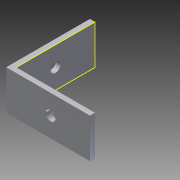
# Autodesk Inventor part: SideSupport
Saved by Autodesk Inventor 2013 (Build 170138000, 138)
## iProperties
Created: 2013-07-15
Part Number: SideSupport
Material: Aluminum 6061
Document SubType Name: Modeling
Designer: root
Density: 1 g/cm^3
Author: root
Autodesk Inventor part; units mm, degrees
ref_plane "YZ Plane" through (0, 0, 0) normal (1, 0, 0) x (0, 1, 0)
ref_plane "XZ Plane" through (0, 0, 0) normal (0, 1, 0) x (-1, 0, 0)
ref_plane "XY Plane" through (0, 0, 0) normal (0, 0, 1) x (1, 0, 0)
sketch "Sketch1" plane through (0, 0, 0) normal (1, 0, 0) x (0, 1, 0)
  line L0 (0, 0) -> (12.7, 0)
  line L1 (12.7, 0) -> (12.7, 25.4)
  line L2 (12.7, 25.4) -> (0, 25.4)
  line L3 (0, 25.4) -> (0, 0)
  dimension "d0" = 25.4
  dimension "d1" = 12.7
  constraints: 8 end point, 2 parallel, 1 horizontal, 1 perpendicular
  measures "d0" distance of L2.end L0.start
  measures "d1" distance of L0.start L0.end
extrude "Extrusion1" add sketch "Sketch1" along normal blind 1.5875
sketch "Sketch2" plane through (1.5875, 0, 0) normal (1, 0, 0) x (0, 0, -1)
  line L0 (0, 0) -> (0, 12.7) projected
  line L1 (0, 12.7) -> (-25.4, 12.7) projected
  line L2 (-25.4, 12.7) -> (-25.4, 0) projected
  line L3 (-25.4, 0) -> (0, 0) projected
sketch "Sketch3" plane through (0, 0, 0) normal (-1, 0, 0) x (0, 0, 1)
  line L0 (25.4, 12.7) -> (26.9875, 12.7)
  line L1 (26.9875, 12.7) -> (26.9875, 0)
  line L2 (26.9875, 0) -> (25.4, 0)
  line L3 (25.4, 0) -> (25.4, 12.7)
  dimension "d4" = 1.5875
  constraints: 8 end point, 2 parallel, 1 horizontal, 1 perpendicular
  measures "d4" distance of L1.end L2.end
extrude "Extrusion2" add sketch "Sketch3" against normal blind 26.9875
sketch "Sketch4" plane through (1.5875, 0, 0) normal (1, 0, 0) x (0, 0, -1)
  line L0 (0, 0) -> (0, 12.7) projected
  line L1 (-25.4, 0) -> (0, 0) projected
  point P0 (-12.7, 6.35)
  dimension "d8" = 6.35
  dimension "d9" = 12.7
  measures "d8" distance from line of L1 point (-12.7, 6.35)
  measures "d9" distance from line of point (-12.7, 6.35) L0
sketch "Sketch5" plane through (26.9875, 12.7, 25.4) normal (0, 0, -1) x (-1, 0, 0)
  line L0 (0, -12.7) -> (0, 0) projected
  line L1 (25.4, -12.7) -> (0, -12.7) projected
  point P0 (26.9875, -12.7)
  point P1 (12.7, -6.35)
  dimension "d10" = 6.35
  dimension "d11" = 12.7
  measures "d10" distance from line of L1 point (12.7, -6.35)
  measures "d11" distance from line of point (12.7, -6.35) L0
hole "Hole1" at (14.2875, 6.35, 25.4) direction (0, 0, 1) diameter 3.175 depth 25.4 tip angle 118
hole "Hole2" at (1.5875, 6.35, 12.7) direction (-1, 0, 0) diameter 3.175 depth 25.4 tip angle 118
body "Solid1"
